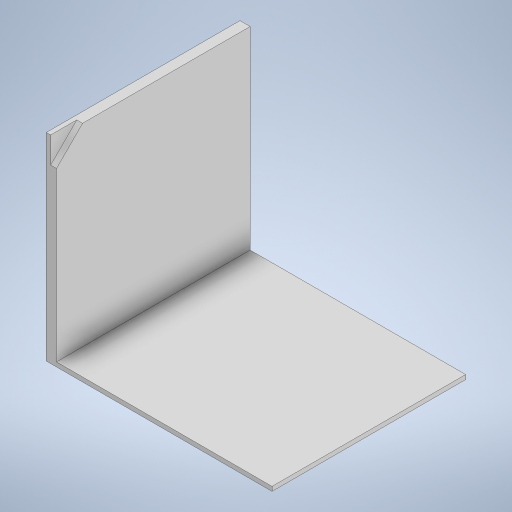
# Autodesk Inventor part: Apple iPad 2022 Hologram
Saved by Autodesk Inventor 2024 (Build 280153000, 153)
## iProperties
Created: 2024-02-23
Part Number: Apple iPad 2022 Hologram
Material: Generic
Document SubType Name: Modeling
Designer: littl
Density: 1 g/cm^3
Appearance: Default
Author: littl
Autodesk Inventor part; units mm, degrees
ref_plane "YZ Plane" through (0, 0, 0) normal (1, 0, 0) x (0, 1, 0)
ref_plane "XZ Plane" through (0, 0, 0) normal (0, 1, 0) x (-1, 0, 0)
ref_plane "XY Plane" through (0, 0, 0) normal (0, 0, 1) x (1, 0, 0)
sketch "Sketch1" plane through (0, 0, 0) normal (0, 1, 0) x (-1, 0, 0)
  line L0 (110, -80) -> (-110, -80)
  line L1 (-110, -80) -> (-110, 80)
  line L2 (-110, 80) -> (110, 80)
  line L3 (110, 80) -> (110, -80)
  line L4 (320.2117, -53.5522) -> (168.036, -53.5522) construction
  line L5 (168.036, -53.5522) -> (168.036, 90.1689) construction
  line L6 (168.036, 90.1689) -> (320.2117, 90.1689) construction
  line L7 (320.2117, 90.1689) -> (320.2117, -53.5522) construction
  line L8 (124.3, -89.75) -> (-124.3, -89.75) construction
  line L9 (-124.3, -89.75) -> (-124.3, 89.75) construction
  line L10 (-124.3, 89.75) -> (124.3, 89.75) construction
  line L11 (124.3, 89.75) -> (124.3, -89.75) construction
  line L12 (124.3, -89.75) -> (-124.3, 89.75) construction
  line L13 (-124.3, -89.75) -> (124.3, 89.75) construction
  line L14 (-152.4, -107.95) -> (152.4, -107.95)
  line L15 (152.4, -107.95) -> (152.4, 107.95)
  line L16 (152.4, 107.95) -> (-152.4, 107.95)
  line L17 (-152.4, 107.95) -> (-152.4, -107.95)
  line L18 (-152.4, -107.95) -> (152.4, 107.95) construction
  line L19 (152.4, -107.95) -> (-152.4, 107.95) construction
  line L20 (177.8, 133.35) -> (177.8, -133.35)
  line L21 (177.8, -133.35) -> (-177.8, -133.35)
  line L22 (-177.8, -133.35) -> (-177.8, 133.35)
  line L23 (-177.8, 133.35) -> (177.8, 133.35)
  point P0 (0, 0)
  dimension "d11" = 220
  dimension "d12" = 160
  dimension "d15" = 248.6
  dimension "d16" = 179.5
  dimension "d18" = 304.8
  dimension "d19" = 215.9
  dimension "d22" = 25.4
  constraints: 40 end point, 8 parallel, 4 midpoint, 4 perpendicular, 3 horizontal, 5 other
  measures "d11" distance of L0.start L0.end
  measures "d12" distance of L0.end L1.end
  measures "d15" distance of L8.start L8.end
  measures "d16" distance of L8.end L9.end
  measures "d18" distance of L14.start L14.end
  measures "d19" distance of L15.end L14.end
  measures "d22" distance between parallel lines of L15 L20
extrude "Top" add sketch "Sketch1" along normal blind 25.4 contours L17 L16 L15 L14 | L20 L21 L22 L23
sketch "Sketch3" plane through (177.8, 0, 133.35) normal (1, 0, 0) x (0, 0, -1)
  line L0 (0, 0) -> (0, 25.4) projected
  line L1 (266.7, 0) -> (266.7, 25.4) projected
  line L2 (0, 0) -> (266.7, 0)
  line L3 (266.7, 0) -> (266.7, -266.7)
  line L4 (266.7, -266.7) -> (0, -266.7)
  line L5 (0, -266.7) -> (0, 0)
  point P0 (133.35, 0)
  dimension "d25" = 266.7
  constraints: 8 end point, 2 parallel, 1 horizontal, 1 perpendicular
  measures "d25" distance between parallel lines of L2 L4
extrude "Right" add sketch "Sketch3" against normal blind 50.8
sketch "Sketch4" plane through (-177.8, 0, -133.35) normal (-1, 0, 0) x (0, 0, 1)
  line L0 (0, 0) -> (0, 25.4) projected
  line L1 (266.7, -266.7) -> (266.7, 0) projected
  line L2 (0, 0) -> (266.7, 0)
  line L3 (266.7, 0) -> (266.7, -266.7)
  line L4 (266.7, -266.7) -> (0, -266.7)
  line L5 (0, -266.7) -> (0, 0)
  point P0 (133.35, 0)
  dimension "d28" = 266.7
  constraints: 8 end point, 2 parallel, 2 perpendicular
  measures "d28" distance of L1.end L3.end
extrude "Left" add sketch "Sketch4" against normal blind 50.8
sketch "Sketch5" plane through (0, 0, 0) normal (1, 0, 0) x (0, 1, 0)
  line L0 (-266.7, -133.35) -> (25.4, -133.35) projected
  line L1 (-266.7, 133.35) -> (-266.7, -133.35) projected
  line L2 (0, -133.35) -> (-266.7, 133.35)
  line L3 (-266.7, 133.35) -> (-275.6803, 124.3697)
  line L4 (-275.6803, 124.3697) -> (-8.9803, -142.3303)
  line L5 (-8.9803, -142.3303) -> (0, -133.35)
  point P0 (0, 0)
  dimension "d31" = 12.7
  constraints: 8 end point, 2 parallel, 1 perpendicular, 1 point on line
  measures "d31" distance of L3.end L1.start
extrude "Plexiglass Cut" cut sketch "Sketch5" along normal mid plane 304.8 contours L4 L1 L2 L0 | L0 L5 L4 | L4 L3 L1
sketch "Sketch6" plane through (-177.8, -266.7, -133.35) normal (0, -1, 0) x (1, 0, 0)
  line L0 (0, 0) -> (0, 266.7) projected
  line L1 (355.6, 0) -> (0, 0) projected
  line L2 (0, 266.7) -> (355.6, 266.7)
  line L3 (355.6, 266.7) -> (355.6, 0)
  line L4 (355.6, 0) -> (0, 0)
  line L5 (0, 0) -> (0, 266.7)
  point P0 (177.8, 133.35)
  constraints: 8 end point, 2 parallel, 1 horizontal, 1 perpendicular
extrude "Bottom" add sketch "Sketch6" along normal blind 25.4
sketch "Sketch9" plane through (0, 25.4, 0) normal (0, 1, 0) x (1, 0, 0)
  line L0 (177.8, -133.35) -> (127, -133.35) projected
  line L1 (177.8, 133.35) -> (-177.8, 133.35) projected
  line L2 (177.8, -133.35) -> (-177.8, -133.35)
  line L3 (-177.8, -133.35) -> (-177.8, 133.35)
  line L4 (-177.8, 133.35) -> (177.8, 133.35)
  line L5 (177.8, 133.35) -> (177.8, -133.35)
  point P0 (0, 0)
  constraints: 8 end point, 2 parallel, 1 horizontal, 1 perpendicular
extrude "Top Flattening" cut sketch "Sketch9" against normal blind 22.4
sketch "Sketch10" plane through (0, 3, 0) normal (0, 1, 0) x (1, 0, 0)
  line L0 (-177.8, -133.35) -> (-177.8, 133.35) projected
  line L1 (-155.4106, 133.35) -> (-177.8, 133.35)
  line L2 (-177.8, 133.35) -> (-177.8, -133.35)
  line L3 (-177.8, -133.35) -> (-155.4106, -133.35)
  line L4 (-155.4106, -133.35) -> (-155.4106, 133.35)
  line L5 (177.8, 133.35) -> (177.8, -133.35)
  line L6 (177.8, -133.35) -> (155.4106, -133.35)
  line L7 (155.4106, -133.35) -> (155.4106, 133.35)
  line L8 (155.4106, 133.35) -> (177.8, 133.35)
  line L9 (152.4, -115.3895) -> (152.4, 133.35) projected
  point P0 (0, 0)
  point P1 (-177.8, 0)
  dimension "d48" = 22.3894
  dimension "d49" = 22.3894
  constraints: 16 end point, 5 parallel, 2 perpendicular, 1 horizontal, 1 midpoint, 1 other
  measures "d48" distance between parallel lines of L4 L0
  measures "d49" distance between parallel lines of L5 L7
extrude "Outer Side Flattening" cut sketch "Sketch10" against normal through all
sketch "Sketch11" plane through (-177.8, -292.1, -133.35) normal (0, -1, 0) x (1, 0, 0)
  line L0 (22.3894, 0) -> (333.2106, 0) projected
  line L1 (333.2106, 0) -> (22.3894, 0)
  line L2 (22.3894, 0) -> (22.3894, 266.7)
  line L3 (22.3894, 266.7) -> (333.2106, 266.7)
  line L4 (333.2106, 266.7) -> (333.2106, 0)
  point P0 (177.8, 133.35)
  constraints: 8 end point, 2 parallel, 1 horizontal, 1 perpendicular
extrude "Bottom Flattening" cut sketch "Sketch11" against normal blind 22.4
sketch "Sketch12" plane through (155.4106, 3, -133.35) normal (0, 0, -1) x (-1, 0, 0)
  line L0 (155.4106, -3) -> (155.4106, -269.7) construction
  line L1 (7.0106, -269.7) -> (7.0106, -3)
  line L2 (7.0106, -3) -> (303.8106, -3)
  line L3 (303.8106, -3) -> (303.8106, -269.7)
  line L4 (303.8106, -269.7) -> (7.0106, -269.7)
  line L5 (7.0106, -269.7) -> (303.8106, -3) construction
  line L6 (7.0106, -3) -> (303.8106, -269.7) construction
  point P0 (155.4106, -136.35)
  point P1 (155.4106, -3)
  dimension "d54" = 296.8
  constraints: 14 end point, 5 midpoint, 3 parallel, 1 perpendicular, 2 other
  measures "d54" distance between parallel lines of L1 L3
extrude "Inner Flattening" cut sketch "Sketch12" against normal through all
sketch "Sketch13" plane through (-155.4106, 3, 133.35) normal (0, 0, 1) x (1, 0, 0)
  line L0 (310.8211, -272.7) -> (310.8211, 0) projected
  line L1 (0, -272.7) -> (0, 0) projected
  line L2 (310.8211, -136.35) -> (0, -136.35)
  line L3 (0, -136.35) -> (0, 0)
  line L4 (0, 0) -> (310.8211, 0)
  line L5 (310.8211, 0) -> (310.8211, -136.35)
  point P0 (155.4106, -3)
  point P1 (310.8211, 0)
  point P2 (0, -136.35)
  constraints: 8 end point, 2 parallel, 1 horizontal, 1 midpoint, 1 perpendicular
extrude "Top Cut" cut sketch "Sketch13" against normal through all
sketch "Sketch14" plane through (-155.4106, -133.35, 133.35) normal (0, 1, 0) x (1, 0, 0)
  line L0 (155.4106, 133.35) -> (0, 133.35)
  line L1 (0, 133.35) -> (0, 266.7)
  line L2 (0, 266.7) -> (155.4106, 266.7)
  line L3 (155.4106, 266.7) -> (155.4106, 133.35)
  line L4 (0, 0) -> (310.8212, 0) projected
  line L5 (0, 266.7) -> (310.8212, 266.7)
  line L6 (310.8212, 266.7) -> (310.8212, 0)
  line L7 (310.8212, 0) -> (0, 0)
  line L8 (0, 0) -> (0, 266.7)
  constraints: 16 end point, 4 parallel, 2 horizontal, 2 perpendicular
extrude "Quarter Cut" cut sketch "Sketch14" against normal through all contours L3 L5 L6 L4 L8 L0
body "Solid1"
